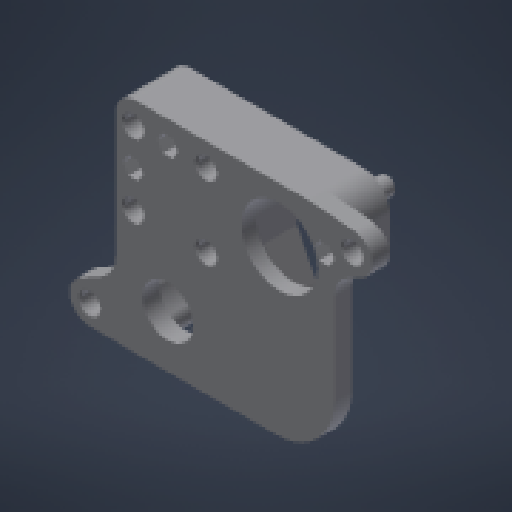
# Autodesk Inventor part: Корпус ноги
Saved by Autodesk Inventor 2025 (Build 290162010, 162A)
## iProperties
Created: 2024-06-21
Part Number: Корпус ноги
Material: Типовые
Document SubType Name: Modeling
Designer: Edward_Higgins
Density: 1 g/cm^3
Appearance: По умолчанию
Mass: 85.3785 g
Surface Area: 299.567 cm^2
Volume: 85.3785 cm^3
Author: Edward_Higgins
Autodesk Inventor part; units mm, degrees
ref_plane "YZ Plane" through (0, 0, 0) normal (1, 0, 0) x (0, 1, 0)
ref_plane "XZ Plane" through (0, 0, 0) normal (0, 1, 0) x (-1, 0, 0)
ref_plane "XY Plane" through (0, 0, 0) normal (0, 0, 1) x (1, 0, 0)
sketch "Эскиз1" plane through (0, 0, 0) normal (0, 0, 1) x (1, 0, 0)
  circle A0 centre (0, 0) radius 4
  circle A1 centre (38.1838, 38.1838) radius 5
  line L0 (38.1838, 38.1838) -> (0, 0) construction
  line L1 (0, 0) -> (58.5741, 0)
  line L2 (48, 57) -> (-11, 57)
  line L3 (-18, 50) -> (-18, -11)
  line L4 (-11, -18) -> (37, -18)
  line L5 (57, 2) -> (57, 48)
  circle A2 centre (0, 0) radius 12.5
  arc A3 (57, 48) -> (48, 57) centre (48, 48) ccw
  arc A4 (-11, 57) -> (-18, 50) centre (-11, 50) ccw
  arc A5 (37, -18) -> (57, 2) centre (37, 2) ccw
  arc A6 (-18, -11) -> (-11, -18) centre (-11, -11) ccw
  point P0 (-11.5166, 0)
  dimension "d0" = 54
  dimension "d1" = 45
  dimension "d2" = 10
  dimension "d8" = 25
  dimension "d37" = 18
  dimension "d38" = 18
  dimension "d39" = 8
  dimension "d86" = 75
  dimension "d87" = 75
  dimension "d88" = 7
  dimension "d89" = 9
  dimension "d90" = 7
  dimension "d91" = 20
  constraints: 12 end point, 8 point on circle, 8 tangent, 7 centre point, 2 coincident, 2 horizontal, 2 parallel, 1 horizontal alignment, 1 perpendicular
  measures "d0" distance of L0.start point (0, 0)
  measures "d1" angle of L1 L0
  measures "d2" diameter of A1
  measures "d8" diameter of A2
  measures "d37" distance from line of L4 point (0, 0)
  measures "d38" distance from line of L3 point (0, 0)
  measures "d39" diameter of A0
  measures "d86" distance between parallel lines of L5 L3
  measures "d87" distance between parallel lines of L2 L4
  measures "d88" radius of A4
  measures "d89" radius of A3
  measures "d90" radius of A6
  measures "d91" radius of A5
extrude "Выдавливание1" add sketch "Эскиз1" against normal blind 5 contours A3 L5 A5 L4 A6 L3 A4 L2
sketch "Эскиз2" plane through (0, 0, -5) normal (0, 0, -1) x (-1, 0, 0)
  line L0 (11.5, 14.5) -> (-35.5, 14.5)
  line L1 (-35.5, 14.5) -> (-35.5, -14.5)
  line L2 (-35.5, -14.5) -> (11.5, -14.5)
  line L3 (11.5, -14.5) -> (11.5, 14.5)
  line L4 (18, -11) -> (18, 50) projected
  arc A0 (11, -18) -> (18, -11) centre (11, -11) ccw projected
  line L5 (-37, -18) -> (11, -18) projected
  line L6 (-42, -11) -> (-42, 11)
  arc A1 (-35, 18) -> (-42, 11) centre (-35, 11) ccw
  line L7 (-35, 18) -> (11, 18)
  arc A2 (18, 11) -> (11, 18) centre (11, 11) ccw
  arc A3 (-42, -11) -> (-35, -18) centre (-35, -11) ccw
  point P0 (0, 0)
  point P1 (11.5, 0)
  dimension "d12" = 29
  dimension "d13" = 47
  dimension "d14" = 11.5
  dimension "d27" = 6.5
  dimension "d28" = 6.5
  dimension "d29" = 3.5
  dimension "d30" = 3.5
  constraints: 12 end point, 6 point on circle, 6 tangent, 3 centre point, 3 equal radius, 2 parallel, 2 perpendicular, 2 point on line, 1 horizontal, 1 horizontal alignment, 1 midpoint, 1 vertical
  measures "d12" distance of L2.end L0.start
  measures "d13" distance of L0.start L0.end
  measures "d14" distance from line of L3 point (0, 0)
  measures "d27" distance between parallel lines of L4 L3
  measures "d28" distance between parallel lines of L6 L1
  measures "d29" distance between parallel lines of L5 L2
  measures "d30" distance between parallel lines of L7 L0
extrude "Выдавливание2" add sketch "Эскиз2" along normal blind 25
sketch "Эскиз3" plane through (0, 0, 0) normal (0, 0, 1) x (1, 0, 0)
  line L0 (48, 57) -> (-11, 57) projected
  arc A0 (-11, 57) -> (-18, 50) centre (-11, 50) ccw projected
  line L1 (-18, 50) -> (-18, -11) projected
  arc A1 (-18, -11) -> (-11, -18) centre (-11, -11) ccw projected
  line L2 (25.1838, 38.1838) -> (25.1838, 17)
  line L3 (25.1838, 17) -> (-18, 17)
  line L4 (-11, -18) -> (37, -18) projected
  arc A2 (37, -18) -> (57, 2) centre (37, 2) ccw projected
  line L5 (57, 2) -> (57, 48) projected
  arc A3 (52.1166, 37.2455) -> (57, 38) centre (54.5, 38) ccw
  line L6 (52.1166, 37.2455) -> (50.5776, 42.1071)
  arc A4 (50.5776, 42.1071) -> (25.1838, 38.1838) centre (38.1838, 38.1838) ccw
  arc A5 (57, 48) -> (48, 57) centre (48, 48) ccw projected
  circle A6 centre (38.1838, 38.1838) radius 5 projected
  point P0 (0, 0)
  point P1 (26.7754, 57)
  dimension "d35" = 13
  dimension "d71" = 40
  dimension "d171" = 19
  constraints: 6 end point, 4 point on circle, 4 tangent, 3 point on line, 2 centre point, 2 coincident, 2 perpendicular
  measures "d35" radius of A4
  measures "d71" distance between parallel lines of L0 L3
  measures "d171" distance from line of L0 A3.centre
extrude "Выдавливание3" add sketch "Эскиз3" along normal blind 13 contours A5 L5 A3 L6 A4 L2 L3 L1 A0 L0
sketch "Эскиз4" plane through (0, 0, 13) normal (0, 0, 1) x (1, 0, 0)
  line L0 (-18, 50) -> (-18, 17) projected
  arc A0 (-11, 57) -> (-18, 50) centre (-11, 50) ccw projected
  line L1 (48, 57) -> (-11, 57) projected
  arc A1 (-11, 57) -> (-18, 50) centre (-11, 50) ccw projected
  line L2 (-18, 50) -> (-18, 17) projected
  line L3 (57, 38) -> (57, 48) projected
  arc A2 (57, 48) -> (48, 57) centre (48, 48) ccw projected
  line L4 (48, 57) -> (-11, 57) projected
  line L5 (-18, 17) -> (25.1838, 17) projected
  line L6 (25.1838, 17) -> (25.1838, 38.1838) projected
  arc A3 (50.5776, 42.1071) -> (25.1838, 38.1838) centre (38.1838, 38.1838) ccw projected
  line L7 (50.5776, 42.1071) -> (52.1166, 37.2455) projected
  arc A4 (52.1166, 37.2455) -> (57, 38) centre (54.5, 38) ccw projected
  line L8 (57, 2) -> (57, 38) projected
  arc A5 (37, -18) -> (57, 2) centre (37, 2) ccw projected
  line L9 (-11, -18) -> (37, -18) projected
  line L10 (-18, 17) -> (-18, -11) projected
  arc A6 (-18, -11) -> (-11, -18) centre (-11, -11) ccw projected
  point P0 (0, 0)
  point P1 (48, 57)
extrude "Выдавливание4" add sketch "Эскиз4" along normal blind 6
sketch "Эскиз5" plane through (0, 0, 19) normal (0, 0, 1) x (1, 0, 0)
  circle A0 centre (0, 0) radius 12.5 projected
  circle A1 centre (0, 0) radius 14
  circle A2 centre (38.1838, 38.1838) radius 5 projected
  circle A3 centre (38.1838, 38.1838) radius 13
  arc A4 (50.5776, 42.1071) -> (25.1838, 38.1838) centre (38.1838, 38.1838) ccw projected
  dimension "d22" = 28
  constraints: 2 coincident, 1 centre point, 3 other
  measures "d22" diameter of A1
extrude "Выдавливание5" cut sketch "Эскиз5" against normal up to surface (6 mm away) contours A0 | A1 | A2 | A3
sketch "Эскиз6" plane through (0, 0, -5) normal (0, 0, -1) x (-1, 0, 0)
  arc A0 (11.5, 4.899) -> (11.5, -4.899) centre (0, 0) ccw projected
  line L0 (11.5, -14.5) -> (11.5, -4.899) projected
  line L1 (11.5, 4.899) -> (11.5, 14.5) projected
  line L2 (11.5, 14.5) -> (-35.5, 14.5) projected
  line L3 (-35.5, 14.5) -> (-35.5, -14.5) projected
  line L4 (-35.5, -14.5) -> (11.5, -14.5) projected
extrude "Выдавливание6" cut sketch "Эскиз6" against normal blind 3
chamfer "Фаска1" distance 1 angle 45 4 edges at (35.5, 14.5, -16) (-11.5, 14.5, -16) (-11.5, -14.5, -16) (35.5, -14.5, -16)
sketch "Эскиз11" plane through (0, 0, 0) normal (0, 0, 1) x (1, 0, 0)
  circle A0 centre (23.9232, 13.7027) radius 9
  circle A1 centre (0, 0) radius 14
  circle A2 centre (38.1838, 38.1838) radius 5 projected
  arc A3 (52.1166, 37.2455) -> (57, 38) centre (54.5, 38) ccw projected
  line L0 (52.1166, 37.2455) -> (50.5776, 42.1071) projected
  arc A4 (50.5776, 42.1071) -> (25.1838, 38.1838) centre (38.1838, 38.1838) ccw projected
  line L1 (25.1838, 38.1838) -> (25.1838, 17) construction
  line L2 (25.1838, 17) -> (-18, 17) construction
  line L3 (-18, 17) -> (-18, -11) projected
  arc A5 (-18, -11) -> (-11, -18) centre (-11, -11) ccw projected
  line L4 (-11, -18) -> (37, -18) projected
  arc A6 (37, -18) -> (57, 2) centre (37, 2) ccw projected
  line L5 (57, 2) -> (57, 38) projected
  circle A7 centre (23.9232, 13.7027) radius 4.0306
  arc A8 (-13.2463, -4.5317) -> (-18, -5.3223) centre (-15.5574, -5.3223) ccw
  arc A9 (-12.1555, -18) -> (-9.2949, -10.4693) centre (-12.1555, -13.6913) ccw
  circle A10 centre (0, 0) radius 14 projected
  point P0 (-11.6477, -17.97)
  dimension "d40" = 18
  constraints: 10 centre point, 6 point on circle, 4 tangent, 2 coincident, 2 point on line, 3 other
  measures "d40" diameter of A0
extrude "Выдавливание7" add sketch "Эскиз11" along normal up to surface (13 mm away) contours A1 A9 A5 L3 A8
fillet "Сопряжение1" radius 6 1 edges at (-18, 17, 6.5)
sketch "Эскиз12" plane through (0, 0, 0) normal (0, 0, 1) x (1, 0, 0)
  circle A0 centre (25.1838, 11.8254) radius 3.5
  line L0 (25.1838, 28.7206) -> (31.9043, 15.1548)
  arc A1 (20.2165, 6.2062) -> (31.9043, 15.1548) centre (25.1838, 11.8254) ccw
  line L1 (20.2165, 6.2062) -> (8.006, 17)
  arc A2 (-11.6477, -17.97) -> (-9.2949, -10.4693) centre (-12.1555, -13.6913) ccw projected
  line L2 (-11, -18) -> (37, -18) projected
  arc A3 (37, -18) -> (57, 2) centre (37, 2) ccw projected
  line L3 (57, 2) -> (57, 38) projected
  arc A4 (52.1166, 37.2455) -> (57, 38) centre (54.5, 38) ccw projected
  line L4 (52.1166, 37.2455) -> (50.5776, 42.1071) projected
  arc A5 (50.5776, 42.1071) -> (25.1838, 38.1838) centre (38.1838, 38.1838) ccw projected
  line L5 (25.1838, 38.1838) -> (25.1838, 17) projected
  line L6 (25.1838, 17) -> (-12, 17) projected
  arc A6 (-18, 23) -> (-12, 17) centre (-12, 23) ccw projected
  line L7 (-18, 23) -> (-18, -5.3223) projected
  arc A7 (-13.2463, -4.5317) -> (-18, -5.3223) centre (-15.5574, -5.3223) ccw projected
  arc A8 (-13.2463, -4.5317) -> (-9.2949, -10.4693) centre (0, 0) ccw projected
  circle A9 centre (0, 0) radius 12.5 projected
  circle A10 centre (38.1838, 38.1838) radius 5 projected
  line L8 (25.1838, 38.1838) -> (25.1838, 17) construction
  arc A11 (-11.6477, -17.97) -> (-11, -18) centre (-11, -11) ccw projected
  point P0 (25.1838, 27.5919)
  point P1 (25.4086, 28.0582)
  dimension "d46" = 7
  dimension "d49" = 4
  constraints: 4 end point, 2 centre point, 2 midpoint, 2 point on circle, 2 point on line, 2 tangent, 1 coincident
  measures "d46" diameter of A0
  measures "d49" radial gap between concentric circles of A1 A0
extrude "Выдавливание8" add sketch "Эскиз12" along normal up to surface (19 mm away) contours A0 | L0 A1 L1 L6 L5
sketch "Эскиз13" plane through (0, 0, -5) normal (0, 0, -1) x (-1, 0, 0)
  circle A0 centre (-38.1838, 38.1838) radius 5 projected
  circle A1 centre (-38.1838, 38.1838) radius 8
  point P0 (0, 0)
  dimension "d50" = 16
  constraints: 1 centre point, 1 coincident
  measures "d50" diameter of A1
extrude "Выдавливание9" add sketch "Эскиз13" along normal blind 9.3
sketch "Эскиз14" plane through (0, 0, 19) normal (0, 0, 1) x (1, 0, 0)
  line L0 (-18, -11) -> (-18, 11) construction
  arc A0 (-11, 18) -> (-18, 11) centre (-11, 11) ccw construction
  line L1 (-11, 18) -> (35, 18) construction
  arc A1 (42, 11) -> (35, 18) centre (35, 11) ccw construction
  line L2 (42, 11) -> (42, -11) construction
  arc A2 (35, -18) -> (42, -11) centre (35, -11) ccw construction
  line L3 (35, -18) -> (-11, -18) construction
  arc A3 (-18, -11) -> (-11, -18) centre (-11, -11) ccw construction
  line L4 (-11.5, 13.5) -> (-11.5, -13.5) construction
  line L5 (-10.5, -14.5) -> (-11.5, -13.5) construction
  line L6 (-10.5, -14.5) -> (34.5, -14.5) construction
  line L7 (35.5, -13.5) -> (34.5, -14.5) construction
  line L8 (35.5, -13.5) -> (35.5, 13.5) construction
  line L9 (34.5, 14.5) -> (35.5, 13.5) construction
  line L10 (34.5, 14.5) -> (-10.5, 14.5) construction
  line L11 (-11.5, 13.5) -> (-10.5, 14.5) construction
  circle A4 centre (0, 0) radius 14 projected
  circle A5 centre (38.1838, 38.1838) radius 13 projected
  line L12 (48, 57) -> (-11, 57) projected
  arc A6 (-11, 57) -> (-18, 50) centre (-11, 50) ccw projected
  line L13 (-18, 50) -> (-18, -11) projected
  arc A7 (-18, -11) -> (-11, -18) centre (-11, -11) ccw projected
  line L14 (-11, -18) -> (37, -18) projected
  arc A8 (37, -18) -> (57, 2) centre (37, 2) ccw projected
  line L15 (57, 2) -> (57, 48) projected
  arc A9 (57, 48) -> (48, 57) centre (48, 48) ccw projected
  circle A10 centre (38.1838, 38.1838) radius 5 projected
  circle A11 centre (0, 0) radius 12.5 projected
  line L16 (25.1838, 28.7206) -> (31.9043, 15.1548) projected
  arc A12 (20.2165, 6.2062) -> (31.9043, 15.1548) centre (25.1838, 11.8254) ccw projected
  line L17 (20.2165, 6.2062) -> (8.006, 17) projected
  line L18 (8.006, 17) -> (-12, 17) projected
  arc A13 (-18, 23) -> (-12, 17) centre (-12, 23) ccw projected
  line L19 (-18, 23) -> (-18, -5.3223) projected
  arc A14 (-13.2463, -4.5317) -> (-18, -5.3223) centre (-15.5574, -5.3223) ccw projected
  arc A15 (-13.2463, -4.5317) -> (-9.2949, -10.4693) centre (0, 0) ccw projected
  arc A16 (-11.6477, -17.97) -> (-9.2949, -10.4693) centre (-12.1555, -13.6913) ccw projected
  line L20 (-11, -18) -> (37, -18) projected
  arc A17 (37, -18) -> (57, 2) centre (37, 2) ccw projected
  line L21 (57, 2) -> (57, 38) projected
  arc A18 (52.1166, 37.2455) -> (57, 38) centre (54.5, 38) ccw projected
  line L22 (52.1166, 37.2455) -> (50.5776, 42.1071) projected
  arc A19 (50.5776, 42.1071) -> (25.1838, 38.1838) centre (38.1838, 38.1838) ccw projected
  line L23 (25.1838, 38.1838) -> (25.1838, 28.7206) projected
  circle A20 centre (13.1838, 24) radius 3.25
  circle A21 centre (-11.8162, 49) radius 3.25
  circle A22 centre (13.1838, 49) radius 3.25
  circle A23 centre (-11.8162, 24) radius 3.25
  circle A24 centre (-26.8162, -11) radius 3.25
  arc A25 (-30.0984, -5.1017) -> (-26.9229, -17.7492) centre (-26.8162, -11) ccw
  line L24 (-30.0984, -5.1017) -> (-18, 1.6306)
  line L25 (-26.9229, -17.7492) -> (-11.1106, -17.9991)
  circle A26 centre (-11.8162, 24) radius 5 construction
  circle A27 centre (13.1838, 24) radius 5 construction
  circle A28 centre (13.1838, 49) radius 5 construction
  circle A29 centre (-11.8162, 49) radius 5 construction
  circle A30 centre (-26.8162, -11) radius 5 construction
  line L26 (48.7429, 56.9693) -> (63.741, 55.727)
  arc A31 (66.0647, 42.8957) -> (63.741, 55.727) centre (63.1838, 49) ccw
  line L27 (66.0647, 42.8957) -> (57, 38.6176)
  circle A32 centre (63.1838, 49) radius 3.25
  arc A33 (57, 48) -> (48, 57) centre (48, 48) ccw projected
  line L28 (57, 2) -> (57, 48) projected
  arc A34 (-11.6477, -17.97) -> (-11, -18) centre (-11, -11) ccw projected
  point P0 (-18, 1.6306)
  point P1 (48.7429, 56.9693)
  dimension "d53" = 6.5
  dimension "d54" = 25
  dimension "d55" = 25
  dimension "d59" = 7
  dimension "d61" = 3.5
  dimension "d62" = 30
  dimension "d70" = 30
  dimension "d103" = 10
  dimension "d104" = 35
  dimension "d105" = 90
  dimension "d107" = 60
  dimension "d108" = 75
  dimension "d109" = 25
  constraints: 13 centre point, 10 equal radius, 8 end point, 7 coincident, 6 point on circle, 6 tangent, 3 horizontal alignment, 2 point on line, 2 vertical alignment
  measures "d53" diameter of A22
  measures "d54" distance of A22.centre A21.centre
  measures "d55" distance of A21.centre A23.centre
  measures "d59" distance from line of L20 A25.centre
  measures "d61" radial gap between concentric circles of A25 A24
  measures "d62" angle of L25 L24
  measures "d70" angle of L27 L26
  measures "d103" diameter of A28
  measures "d104" vertical distance of A24.centre A23.centre
  measures "d105" horizontal distance of A24.centre A31.centre
  measures "d107" vertical distance of A24.centre A31.centre
  measures "d108" distance of A21.centre A31.centre
  measures "d109" horizontal distance of A31.centre A5.centre
extrude "Выдавливание10" cut sketch "Эскиз14" against normal up to surface (24 mm away) contours A20 | A21 | A22 | A23 | A24
extrude "Выдавливание11" add sketch "Эскиз14" against normal up to surface (6 mm away) contours L13 A7 L25 A25 L24 | L26 A31 L27 L15 A9
fillet "Сопряжение2" radius 3 8 edges at (39.9497, 15.9497, -30) (42, 0, -30) (39.9497, -15.9497, -30) (12, -18, -30) (-15.9497, -15.9497, -30) (-18, 0, -30) (-15.9497, 15.9497, -30) (12, 18, -30)
fillet "Сопряжение3" radius 5 6 edges at (39.9497, 15.9497, -5) (12, 18, -5) (-15.9497, 15.9497, -5) (39.9497, -15.9497, -5) (42, 0, -5) (46.1838, 38.1838, -5)
sketch "Эскиз15" plane through (0, 0, -5) normal (0, 0, -1) x (-1, 0, 0)
  arc A0 (-10.0914, 23) -> (-16.2761, 23) centre (-13.1838, 24) ccw projected
  arc A1 (14.6608, 22.428) -> (8.7239, 23) centre (11.8162, 24) ccw projected
  circle A2 centre (-13.1838, 24) radius 5.5
  circle A3 centre (11.8162, 24) radius 5.5
  point P0 (0, 0)
  point P1 (7.7635, 25)
  point P2 (14.2475, 24.8317)
  dimension "d74" = 11
  constraints: 2 centre point, 2 coincident, 1 equal radius
  measures "d74" diameter of A2
extrude "Выдавливание12" cut sketch "Эскиз15" along normal blind 10
chamfer "Фаска2" distance 2 angle 45 2 edges at (35.5, 0, -30) (-11.5, 0, -30)
chamfer "Фаска3" distance 0.5 angle 45 17 edges at (9.9338, 49, -5) (-15.0662, 49, -5) (-12.628, 27.147, -5) (-11.5045, 20.765, -5) (-8.6059, 23.4938, -5) (16.3941, 23.4938, -5) (13.1838, 20.75, -5) (12.6776, 27.2103, -5) (43.1838, 38.1838, -14.3) (33.1838, 38.1838, 0) (-30.0662, -11, 19) (59.9338, 49, 19) (9.9338, 49, 19) (9.9338, 24, 19) (-15.0662, 24, 19) (-15.0662, 49, 19) (-30.0662, -11, 13)
chamfer "Фаска4" distance 1 angle 45 2 edges at (51.0313, 40.1687, 13) (38.1838, 25.1838, 13)
fillet "Сопряжение4" [suppressed]
fillet "Сопряжение5" [suppressed]
fillet "Сопряжение6" radius 1 10 edges at (54.364, 54.364, -5) (57, 25, -5) (54.0186, -8.5055, -5) (43.9725, -16.7452, -5.1845) (39.3392, -17.8627, -6.847) (35.9926, -18, -9.1661) (-15.9497, 54.9497, -5) (-18, 35.3734, -5) (-18, 15.4624, -6.6354) (18.5, 57, -5)
fillet "Сопряжение7" radius 9.25 2 edges at (57, 38.6176, 16) (-18, 1.6306, 16)
sketch "Эскиз16" plane through (-10.5, 14.5, -30) normal (0, -1, 0) x (1, 0, 0)
  circle A0 centre (14.5, 5) radius 1 projected
  circle A1 centre (14.5, 17) radius 1 projected
  circle A2 centre (38.5, 5) radius 1 projected
  circle A3 centre (38.5, 17) radius 1 projected
  line L0 (43.75, 28) -> (1.25, 28) projected
  line L1 (43.75, 28) -> (43.75, -6) projected
  line L2 (1.25, -6) -> (43.75, -6) projected
  line L3 (1.25, 28) -> (1.25, -6) projected
  point P0 (10.5, 30)
extrude "Выдавливание13" cut sketch "Эскиз16" along normal mid plane 92.5 contours A0 | A1 | A2 | A3
sketch "Эскиз18" plane through (-11, 18, -27) normal (0, 1, 0) x (1, 0, 0)
  circle A0 centre (15, -2) radius 1 projected
  circle A1 centre (15, -14) radius 1 projected
  circle A2 centre (39, -2) radius 1 projected
  circle A3 centre (39, -14) radius 1 projected
  circle A4 centre (15, -14) radius 2.5
  circle A5 centre (15, -2) radius 2.5
  circle A6 centre (39, -2) radius 2.5
  circle A7 centre (39, -14) radius 2.5
  point P0 (11, -27)
  dimension "d113" = 5
  constraints: 4 centre point, 4 coincident, 3 equal radius
  measures "d113" diameter of A5
extrude "Выдавливание14" cut sketch "Эскиз18" against normal blind 1 contours A0 | A1 | A2 | A3 | A4 | A5 | A6 | A7
ref_plane "РабПлоскость1" through (-10.5, 0, -30) normal (0, 1, 0) x (1, 0, 0)
mirror "Зеркальное отражение1" about plane through (-10.5, 0, -30) normal (0, 1, 0) of "Выдавливание14"
sketch "Эскиз19" plane through (0, 0, 0) normal (0, 0, 1) x (1, 0, 0)
  line L0 (92.3303, 73.4893) -> (-53.1485, 73.4893)
  line L1 (-53.1485, 73.4893) -> (-53.1485, -32.6202)
  line L2 (-53.1485, -32.6202) -> (92.3303, -32.6202)
  line L3 (92.3303, -32.6202) -> (92.3303, 73.4893)
  point P0 (0, 0)
  constraints: 8 end point, 2 parallel, 1 horizontal, 1 perpendicular
extrude "Выдавливание15" cut sketch "Эскиз19" against normal up to surface (30 mm away)
sketch "Эскиз20" plane through (0, 0, 0) normal (0, 0, -1) x (-1, 0, 0)
  circle A0 centre (-0.6838, 36.5) radius 8
  circle A1 centre (-25.1838, 11.8254) radius 4.5
  circle A2 centre (12.7279, -12.7279) radius 3
  circle A3 centre (-50.9117, 50.9117) radius 3
  circle A4 centre (11.8162, 49) radius 3.25 projected
  circle A5 centre (11.8162, 24) radius 3.25 projected
  circle A6 centre (-13.1838, 24) radius 3.25 projected
  circle A7 centre (-13.1838, 49) radius 3.25 projected
  arc A8 (-31.9043, 15.1548) -> (-20.2165, 6.2062) centre (-25.1838, 11.8254) ccw projected
  line L0 (-20.2165, 6.2062) -> (-8.006, 17) projected
  line L1 (-8.006, 17) -> (12, 17) projected
  arc A9 (12, 17) -> (18, 23) centre (12, 23) ccw projected
  line L2 (18, 50) -> (18, 23) projected
  arc A10 (18, 50) -> (11, 57) centre (11, 50) ccw projected
  line L3 (-48, 57) -> (11, 57) projected
  arc A11 (-48, 57) -> (-57, 48) centre (-48, 48) ccw projected
  line L4 (-57, 38) -> (-57, 48) projected
  arc A12 (-57, 38) -> (-52.1166, 37.2455) centre (-54.5, 38) ccw projected
  line L5 (-52.1166, 37.2455) -> (-50.5776, 42.1071) projected
  arc A13 (-25.1838, 38.1838) -> (-50.5776, 42.1071) centre (-38.1838, 38.1838) ccw projected
  line L6 (-25.1838, 38.1838) -> (-25.1838, 28.7206) projected
  line L7 (-25.1838, 28.7206) -> (-31.9043, 15.1548) projected
  line L8 (-13.1838, 49) -> (11.8162, 24) construction
  line L9 (-13.1838, 24) -> (11.8162, 49) construction
  line L10 (-50.9117, 50.9117) -> (12.7279, -12.7279) construction
  point P0 (0, 0)
  point P1 (-0.6838, 36.5)
  dimension "d118" = 16
  dimension "d119" = 9
  dimension "d120" = 6
  dimension "d121" = 6
  dimension "d123" = 18
  dimension "d124" = 18
  constraints: 6 end point, 4 centre point, 2 coincident, 2 midpoint, 2 point on line
  measures "d118" diameter of A0
  measures "d119" diameter of A1
  measures "d120" diameter of A3
  measures "d121" diameter of A2
  measures "d123" distance of A13.centre L10.start
  measures "d124" distance of L10.end point (0, 0)
extrude "Выдавливание16" add sketch "Эскиз20" along normal blind 5 contours A0 | A3
sketch "Эскиз21" plane through (0, 0, 13) normal (0, 0, -1) x (-1, 0, 0)
  circle A0 centre (0, 0) radius 14 projected
extrude "Выдавливание18" add sketch "Эскиз21" against normal up to surface (6 mm away)
sketch "Эскиз22" plane through (0, 0, 13) normal (0, 0, -1) x (-1, 0, 0)
  circle A0 centre (0, 0) radius 8.65
  circle A1 centre (0, 0) radius 12.65
  dimension "d131" = 17.3
  dimension "d132" = 4
  constraints: 2 centre point, 2 coincident
  measures "d131" diameter of A0
  measures "d132" radial gap between concentric circles of A0 A1
extrude "Выдавливание20" cut sketch "Эскиз22" against normal blind 9.25 contours A0
sketch "Эскиз23" plane through (0, 0, 19) normal (0, 0, 1) x (1, 0, 0)
  circle A0 centre (46.4974, -10.4693) radius 1.75
  arc A1 (37, -18) -> (57, 2) centre (37, 2) ccw projected
  circle A2 centre (0, 49) radius 1.75
  circle A3 centre (-11.8162, 36.5) radius 1.75
  circle A4 centre (53.5, 44) radius 1.75
  arc A5 (57, 48) -> (48, 57) centre (48, 48) ccw projected
  line L0 (57, 38) -> (57, 48) projected
  arc A6 (52.1166, 37.2455) -> (57, 38) centre (54.5, 38) ccw projected
  line L1 (52.1166, 37.2455) -> (50.5776, 42.1071) projected
  arc A7 (50.5776, 42.1071) -> (25.1838, 38.1838) centre (38.1838, 38.1838) ccw projected
  line L2 (48, 57) -> (-11, 57) projected
  line L3 (-18, 50) -> (-18, 23) projected
  arc A8 (-13.2463, -4.5317) -> (-9.2949, -10.4693) centre (0, 0) ccw projected
  arc A9 (-11.6477, -17.97) -> (-9.2949, -10.4693) centre (-12.1555, -13.6913) ccw projected
  arc A10 (-18, -11) -> (-11.6477, -17.97) centre (-11, -11) ccw projected
  line L4 (-18, -5.3223) -> (-18, -11) projected
  circle A11 centre (-11.8162, 49) radius 3.25 projected
  circle A12 centre (13.1838, 49) radius 3.25 projected
  circle A13 centre (-11.8162, 24) radius 3.25 projected
  line L5 (-18, -5.3223) -> (-18, -11) projected
  arc A14 (-13.2463, -4.5317) -> (-18, -5.3223) centre (-15.5574, -5.3223) ccw projected
  arc A15 (-13.2463, -4.5317) -> (-9.2949, -10.4693) centre (0, 0) ccw projected
  arc A16 (-11.6477, -17.97) -> (-9.2949, -10.4693) centre (-12.1555, -13.6913) ccw projected
  arc A17 (-18, -11) -> (-11.6477, -17.97) centre (-11, -11) ccw projected
  line L6 (-1.7321, 52) -> (1.7321, 52)
  line L7 (1.7321, 52) -> (3.4641, 49)
  line L8 (3.4641, 49) -> (1.7321, 46)
  line L9 (1.7321, 46) -> (-1.7321, 46)
  line L10 (-1.7321, 46) -> (-3.4641, 49)
  line L11 (-3.4641, 49) -> (-1.7321, 52)
  line L12 (-13.5483, 39.5) -> (-10.0842, 39.5)
  line L13 (-10.0842, 39.5) -> (-8.3521, 36.5)
  line L14 (-8.3521, 36.5) -> (-10.0842, 33.5)
  line L15 (-10.0842, 33.5) -> (-13.5483, 33.5)
  line L16 (-13.5483, 33.5) -> (-15.2803, 36.5)
  line L17 (-15.2803, 36.5) -> (-13.5483, 39.5)
  line L18 (51.7679, 47) -> (55.2321, 47)
  line L19 (55.2321, 47) -> (56.9641, 44)
  line L20 (56.9641, 44) -> (55.2321, 41)
  line L21 (55.2321, 41) -> (51.7679, 41)
  line L22 (51.7679, 41) -> (50.0359, 44)
  line L23 (50.0359, 44) -> (51.7679, 47)
  line L24 (44.7654, -7.4693) -> (48.2295, -7.4693)
  line L25 (48.2295, -7.4693) -> (49.9615, -10.4693)
  line L26 (49.9615, -10.4693) -> (48.2295, -13.4693)
  line L27 (48.2295, -13.4693) -> (44.7654, -13.4693)
  line L28 (44.7654, -13.4693) -> (43.0333, -10.4693)
  line L29 (43.0333, -10.4693) -> (44.7654, -7.4693)
  point P0 (51.1421, -12.1421)
  point P1 (-18, 36.5)
  dimension "d137" = 3.5
  dimension "d162" = 6
  dimension "d166" = 13
  dimension "d167" = 3.5
  constraints: 48 end point, 4 centre point, 4 coincident, 4 horizontal, 3 equal length, 3 equal radius, 2 horizontal alignment, 2 vertical alignment, 1 midpoint, 1 point on circle, 52 other
  measures "d137" diameter of A0
  measures "d162" distance between parallel lines of L21 L18
  measures "d166" distance from line of A4.centre L2
  measures "d167" distance from line of L0 A4.centre
extrude "Выдавливание21" cut sketch "Эскиз23" against normal up to surface (24 mm away) contours A2 | A3 | A4
extrude "Выдавливание27" cut sketch "Эскиз23" against normal blind 7 contours A2 | A3 | A4 | L6 L7 L8 L9 L10 L11 | L12 L13 L14 L15 L16 L17 | L18 L19 L20 L21 L22 L23
chamfer "Фаска5" distance 0.8 angle 45 7 edges at (51.75, 44, 0) (-1.75, 49, 0) (-13.5662, 36.5, 0) (9.9338, 49, 0) (-15.0662, 49, 0) (-15.0662, 24, 0) (9.9338, 24, 0)
equation "\"d38\" = d37"
equation "\"d28\" = d27"
equation "\"d30\" = d29"
